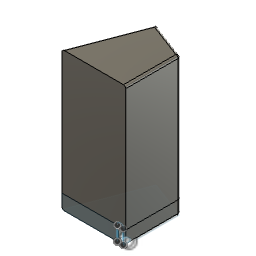
AC Shroud (5 gang) v3 (Autodesk Fusion 360 design; units mm, degrees)
Autodesk Fusion 360 part; units mm, degrees
sketch "Sketch1" plane through (0, 0, 0) normal (0, 1, 0) x (1, 0, 0)
  line L0 (0, 0) -> (140, 0)
  line L1 (140, 0) -> (139.971, 118.0157)
  line L2 (56.8683, 149.5527) -> (0, 0)
  line L3 (10.3074, 27.1064) -> (50.1152, 131.7933)
  line L4 (10.3074, 27.1064) -> (73.1475, 3.2111)
  line L5 (50.1152, 131.7933) -> (62.2663, 127.1727)
  line L6 (62.2663, 127.1727) -> (22.4585, 22.4859)
  line L7 (56.8683, 149.5527) -> (59.6929, 148.5419)
  line L8 (58.5187, 145.4746) -> (52.9119, 130.7298)
  line L9 (4.2368, 2.7013) -> (13.1115, 26.0401)
  line L10 (-137, 154.5) -> (-92, 154.5)
  line L11 (-37, 139.5) -> (-37, 79.5)
  line L12 (-92, 64.5) -> (-137, 64.5)
  line L13 (-37, 109.5) -> (-37, 139.5)
  line L14 (-37, 109.5) -> (-37, 79.5)
  line L15 (-137, 154.5) -> (-92, 154.5)
  line L16 (-92, 64.5) -> (-137, 64.5)
  line L17 (-137, 64.5) -> (-137, 154.5)
  line L18 (-37, 139.5) -> (-92, 154.5)
  line L19 (-37, 79.5) -> (-92, 64.5)
  line L20 (4.2368, 2.7013) -> (137.5, 2.5)
  line L21 (73.1475, 3.2111) -> (74.7683, 2.5948)
  line L22 (59.6929, 148.5419) -> (117.2158, 126.6684)
  line L23 (117.2158, 126.6684) -> (139.971, 118.0157)
  line L24 (58.5187, 145.4746) -> (137.5, 115.4415)
  line L25 (137.5, 115.4415) -> (137.5, 2.5)
  line L26 (46.2055, 121.5115) -> (58.3566, 116.891)
  dimension "d1" = 140
  dimension "d4" = 160
  dimension "d5" = 29
  dimension "d6" = 112
  dimension "d7" = 13
  constraint coincident L0.start L2.end
  constraint horizontal L0
  constraint parallel L2 L3
  constraint perpendicular L3 L4
  constraint perpendicular L3 L5
  constraint coincident L4 L6.end
  constraint perpendicular L4 L6
  constraint coincident L5 L8.end
  constraint perpendicular L5 L8
  constraint coincident L4 L9.end
  constraint perpendicular L4 L9
  constraint horizontal L10
  constraint vertical L11
  constraint horizontal L12
  constraint parallel L11 L13
  constraint parallel L11 L14
  constraint horizontal L15
  constraint horizontal L16
  constraint vertical L17
  constraint coincident L11 L13.start
  constraint coincident L20 L21.end
  constraint perpendicular L8 L22
  constraint perpendicular L8 L23
  constraint perpendicular L8 L24
  constraint coincident L6 L26.end
  constraint perpendicular L6 L26
  measures "d1" distance of L0.start L0.end
  measures "d4" distance of L2.start L0.start
  measures "d5" distance of L0.start L3.start
  measures "d6" distance of L3.start L3.end
  measures "d7" distance of L3.end L5.end
extrude "Extrude1" add sketch "Sketch1" along normal blind 270 contours L0 L1 L2 L4 L5 L7 L8 L9 L20 L22 L23 L24 L25 | L2 L3 L4 L6 L26 | L2 L3 L5 L6 L26 | L4 L9 L20 L21 makes body 1
sketch "Sketch2" plane through (0, 270, 0) normal (0, 1, 0) x (-1, 0, 0)
  line L0 (-52.9119, -130.7298) -> (-58.5187, -145.4746)
  line L1 (-58.5187, -145.4746) -> (-137.5, -115.4415)
  line L2 (-137.5, -115.4415) -> (-137.5, -2.5)
  line L3 (-137.5, -2.5) -> (-74.7683, -2.5948)
  line L4 (-74.7683, -2.5948) -> (-22.4585, -22.4859)
  line L5 (-22.4585, -22.4859) -> (-62.2663, -127.1727)
  line L6 (-62.2663, -127.1727) -> (-52.9119, -130.7298)
  line L7 (-56.8683, -149.5527) -> (0, 0)
  line L8 (0, 0) -> (-140, 0)
  line L9 (-140, 0) -> (-139.971, -118.0157)
  line L10 (-139.971, -118.0157) -> (-59.6929, -148.5419)
  line L11 (-59.6929, -148.5419) -> (-56.8683, -149.5527)
  line L12 (-140, 0) -> (-139.971, -118.0157)
  line L13 (0, 0) -> (-140, 0)
  line L14 (-10.3074, -27.1064) -> (-50.1152, -131.7933)
  line L15 (-59.6929, -148.5419) -> (-117.2158, -126.6684)
  line L16 (-56.8683, -149.5527) -> (0, 0)
extrude "Extrude2" add sketch "Sketch2" along normal blind 3 contours L0 L1 L2 L3 L4 L5 L6 | L7 L8 L9 L10 L11 L12 L13 L14 L15 L16 bodies 1
extrude "Extrude3" cut sketch "Sketch1" along normal blind 245 contours L2 L3 L4 L6 L26 bodies 1
extrude "Extrude4" add sketch "Sketch1" against normal blind 28 separate body contours L0 L1 L2 L4 L5 L7 L8 L9 L20 L22 L23 L24 L25 | L2 L3 L4 L6 L26 | L2 L3 L5 L6 L26 | L4 L9 L20 L21 makes body 2
sketch "Sketch3" plane through (0, -28, 0) normal (0, -1, 0) x (1, 0, 0)
  line L0 (58.5187, -145.4746) -> (52.9119, -130.7298)
  line L1 (52.9119, -130.7298) -> (62.2663, -127.1727)
  line L2 (62.2663, -127.1727) -> (22.4585, -22.4859)
  line L3 (22.4585, -22.4859) -> (74.7683, -2.5948)
  line L4 (74.7683, -2.5948) -> (137.5, -2.5)
  line L5 (137.5, -2.5) -> (137.5, -115.4415)
  line L6 (137.5, -115.4415) -> (58.5187, -145.4746)
  line L7 (0, 0) -> (56.8683, -149.5527)
  line L8 (56.8683, -149.5527) -> (59.6929, -148.5419)
  line L9 (59.6929, -148.5419) -> (139.971, -118.0157)
  line L10 (139.971, -118.0157) -> (140, 0)
  line L11 (140, 0) -> (0, 0)
  line L12 (140, 0) -> (139.971, -118.0157)
  line L13 (59.6929, -148.5419) -> (117.2158, -126.6684)
  line L14 (10.3074, -27.1064) -> (50.1152, -131.7933)
  line L15 (0, 0) -> (140, 0)
  line L16 (56.8683, -149.5527) -> (0, 0)
  line L17 (117.2158, -126.6684) -> (139.971, -118.0157)
  line L18 (56.8683, -149.5527) -> (59.6929, -148.5419)
extrude "Extrude5" add sketch "Sketch3" along normal blind 3 contours L0 L1 L2 L3 L4 L5 L6 | L7 L8 L9 L10 L11 L12 L13 L14 L15 L16 L17 L18 bodies 2
sketch "Sketch4" plane through (0, 0, 0) normal (0, 0, 1) x (1, 0, 0)
  line L0 (140, 0) -> (0, 0)
  line L1 (0, 0) -> (0, -31)
  line L2 (0, -31) -> (140, -31)
  line L3 (140, -31) -> (140, 0)
  line L4 (134.5, 0) -> (134.5, -31)
  line L5 (121.5, 0) -> (121.5, -31)
  arc A0 (134.5, 0) -> (121.5, 0) centre (128, 0) ccw
  dimension "d28" = 13
  constraint coincident L0 A0.centre
  constraint coincident L0 L4.start
  constraint coincident L2 L4.end
  constraint perpendicular L2 L4
  constraint coincident L0 L5.start
  constraint coincident L2 L5.end
  constraint perpendicular L2 L5
  measures "d28" diameter of A0
sketch "Sketch5" plane through (0, -31, 0) normal (0, -1, 0) x (1, 0, 0)
  line L0 (0, 0) -> (56.8683, -149.5527)
  line L1 (56.8683, -149.5527) -> (59.6929, -148.5419)
  line L2 (59.6929, -148.5419) -> (139.971, -118.0157)
  line L3 (139.971, -118.0157) -> (140, 0)
  line L4 (140, 0) -> (0, 0)
  line L5 (121.5, 0) -> (121.5, -12.5)
  line L6 (134.461, -12.5032) -> (134.461, 0)
  arc A0 (121.5, -12.5) -> (134.461, -12.5) centre (127.9805, -12.5016) ccw
  constraint coincident L4 L5.start
  constraint perpendicular L4 L5
  constraint coincident L4 L6.end
  constraint perpendicular L4 L6
  constraint coincident L6 A0.end
extrude "Extrude6" cut sketch "Sketch5" against normal blind 3 contours L4 L5 L6 A0 bodies 2
extrude "Extrude7" cut sketch "Sketch4" against normal blind 3 contours L0 L2 L4 L5 | L0 A0 bodies 2
extrude "Extrude8" cut sketch "Sketch4" against normal blind 3 contours L0 A0 bodies 1
sketch "Sketch7" plane through (0, -28, 0) normal (0, 1, 0) x (-1, 0, 0)
  line L0 (-134.461, -3) -> (-134.5, -3)
  line L1 (-134.5, -3) -> (-134.5, -2.5045)
  line L2 (-134.5, -2.5045) -> (-137.5, -2.5)
  line L3 (-137.5, -2.5) -> (-137.5, -115.4415)
  line L4 (-137.5, -115.4415) -> (-58.5187, -145.4746)
  line L5 (-58.5187, -145.4746) -> (-52.9119, -130.7298)
  line L6 (-52.9119, -130.7298) -> (-62.2663, -127.1727)
  line L7 (-62.2663, -127.1727) -> (-22.4585, -22.4859)
  line L8 (-22.4585, -22.4859) -> (-74.7683, -2.5948)
  line L9 (-74.7683, -2.5948) -> (-121.5, -2.5242)
  line L10 (-121.5, -2.5242) -> (-121.5, -12.5)
  arc A0 (-134.461, -12.5) -> (-121.5, -12.5) centre (-127.9805, -12.5016) ccw
  line L11 (-134.461, -12.5) -> (-134.461, -3)
  line L12 (-58.5187, -145.4746) -> (-52.9119, -130.7298)
  line L13 (-52.9119, -130.7298) -> (-62.2663, -127.1727)
  line L14 (-62.2663, -127.1727) -> (-67.8731, -141.9175)
  line L15 (-67.8731, -141.9175) -> (-58.5187, -145.4746)
  line L16 (-137.5, -115.4415) -> (-118.8059, -122.55)
  line L17 (-137.5, -115.4415) -> (-137.5, -95.4415)
  line L18 (-118.8059, -122.55) -> (-137.5, -95.4415)
  line L19 (-64.5445, -6.4824) -> (-94.5445, -6.4824)
  line L20 (-94.5445, -6.4824) -> (-104.888, -2.5493)
  dimension "d35" = 20
  dimension "d36" = 20
  dimension "d37" = 30
  constraint perpendicular L12 L13
  constraint parallel L12 L14
  constraint parallel L13 L15
  constraint coincident L5.end L6.start
  constraint perpendicular L6 L12
  constraint coincident L4.end L5.start
  constraint coincident L3.end L4.start
  constraint parallel L4 L16
  constraint parallel L3 L17
  constraint coincident L8 L19.start
  constraint horizontal L19
  constraint coincident L9 L20.end
  constraint parallel L8 L20
  measures "d35" distance of L3.end L16.end
  measures "d36" distance of L3.end L17.end
  measures "d37" distance of L19.start L19.end
extrude "Extrude9" add sketch "Sketch7" along normal blind 27.5 contours L3 L4 L16 L17 L18 | L8 L9 L19 L20 | L4 L5 L6 L12 L13 L14 L15 bodies 2
extrude "Extrude10" add 3 faces at (62.8861, -0.5, -138.1883) (131.2686, -0.5, -111.1443) (91.4002, -0.5, -3.8755) along direction (0, 1, 0) blind 10 draft -5 on bodies 2 bodies 2
fillet "Fillet1" radius 5 5 edges at (28.4341, 273, -74.7763) (56.8683, 136.5, -149.5527) (99.8319, 273, -133.2788) (139.9855, 273, -59.0078) (139.971, 136.5, -118.0157) on bodies 1
fillet "Fillet2" radius 5 5 edges at (56.8683, -15.5, -149.5527) (139.971, -15.5, -118.0157) (139.9855, -31, -59.0078) (99.8319, -31, -133.2788) (28.4341, -31, -74.7763) on bodies 2
fillet "Fillet3" radius 3 7 edges at (98.0094, 270, -130.4581) (137.5, 270, -58.9708) (106.1341, 270, -2.5474) (48.6134, 270, -12.5403) (55.7153, 270, -138.1022) (42.3624, 270, -74.8293) (57.5891, 270, -128.9513) on bodies 1
fillet "Fillet4" radius 3 9 edges at (43.5015, -28, -14.4842) (45.1658, -28, -82.2017) (79.5445, -28, -6.4824) (99.7162, -28, -4.5159) (113.194, -28, -2.5367) (136, -28, -2.5023) (137.5, -28, -48.9708) (128.153, -28, -108.9958) (93.3395, -28, -132.2338) on bodies 2
